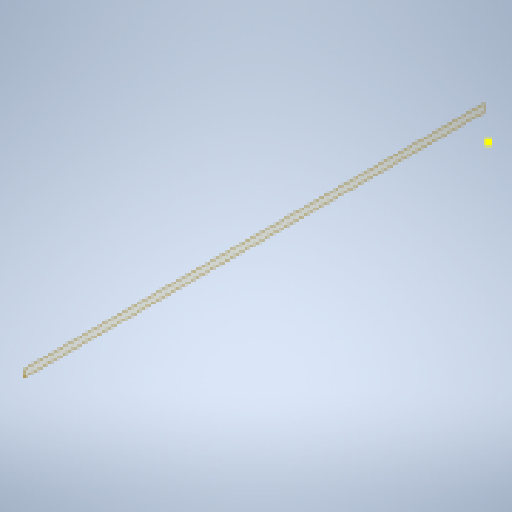
# Autodesk Inventor part: крепёж_мотора
Saved by Autodesk Inventor 2023 (Build 270158000, 158)
## iProperties
Created: 2025-12-12
Part Number: крепёж_мотора
Material: Типовые
Document SubType Name: Modeling
Designer: garin
Density: 1 g/cm^3
Appearance: По умолчанию
Author: garin
Autodesk Inventor part; units mm, degrees
ref_plane "YZ Plane" through (0, 0, 0) normal (1, 0, 0) x (0, 1, 0)
ref_plane "XZ Plane" through (0, 0, 0) normal (0, 1, 0) x (-1, 0, 0)
ref_plane "XY Plane" through (0, 0, 0) normal (0, 0, 1) x (1, 0, 0)
ref_plane "РабПлоскость1" through (57.3886, 15.9976, 24.7396) normal (1, 0, 0) x (0, 1, 0)
sketch "Эскиз1" plane through (57.3886, 15.9976, 24.7396) normal (1, 0, 0) x (0, 1, 0)
  line L0 (-3, 27.5) -> (-3, 52.5)
  circle A0 centre (-16.5, 48) radius 1.5
  circle A1 centre (-16.5, 31) radius 1.5
  circle A2 centre (-16.5, 40) radius 4
  line L1 (-3, 52.5) -> (-3, 27.5)
  line L2 (-31, 54) -> (-3, 54)
  line L3 (-3, 54) -> (-3, 40)
  line L4 (-3, 54) -> (-31, 54)
  line L5 (-31, 54) -> (-31, 26)
  line L6 (-31, 26) -> (-3, 26)
  line L7 (-3, 26) -> (-3, 54)
  circle A3 centre (-16.5, 40) radius 12.75
  point P0 (-15.9976, -24.7396)
  dimension "d12" = 28
  dimension "d15" = 25.5
  constraints: 16 end point, 4 centre point, 3 equal length, 1 coincident, 1 horizontal, 1 midpoint, 1 perpendicular
  measures "d12" distance of L2.start L2.end
  measures "d15" diameter of A3
extrude "Выдавливание1" add sketch "Эскиз1" against normal blind 3 contours A3
